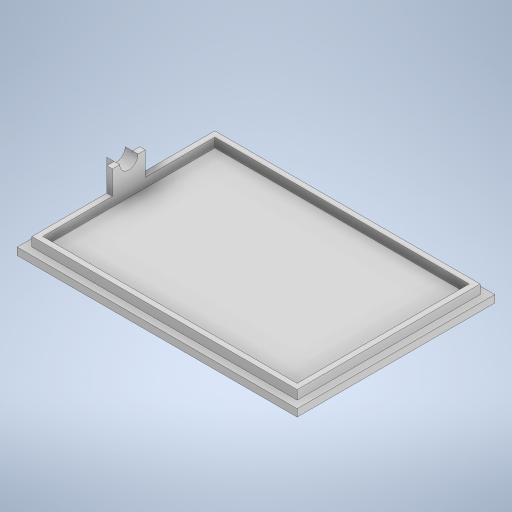
# Autodesk Inventor part: Golf Cart Mainboard Lid
Saved by Autodesk Inventor 2024 (Build 280153000, 153)
## iProperties
Created: 2023-08-08
Part Number: Golf Cart Mainboard Lid
Material: Generic
Document SubType Name: Modeling
Designer: techn
Density: 1 g/cm^3
Appearance: Default
Author: techn
## iProperties of the stored document Golf Cart Mainboard Lid_3DPrint.ipt
Created: 2023-08-08
Part Number: Golf Cart Mainboard Lid_3DPrint
Material: Generic
Document SubType Name: Modeling
Designer: techn
Density: 1 g/cm^3
Appearance: Default
Author: techn
Autodesk Inventor part; units mm, degrees
ref_plane "YZ Plane" through (0, 0, 0) normal (1, 0, 0) x (0, 1, 0)
ref_plane "XZ Plane" through (0, 0, 0) normal (0, 1, 0) x (-1, 0, 0)
ref_plane "XY Plane" through (0, 0, 0) normal (0, 0, 1) x (1, 0, 0)
sketch "Sketch1" plane through (0, 0, 0) normal (0, 1, 0) x (-1, 0, 0)
  line L0 (0, 0) -> (-153, 0)
  line L1 (-153, 0) -> (-153, 108)
  line L2 (-153, 108) -> (0, 108)
  line L3 (0, 108) -> (0, 0)
  dimension "d0" = 153
  dimension "d1" = 108
  constraints: 8 end point, 2 parallel, 1 horizontal, 1 perpendicular
  measures "d0" distance of L1.end L2.end
  measures "d1" distance of L0.end L1.end
extrude "Extrusion1" add sketch "Sketch1" along normal blind 4
sketch "Sketch2" plane through (0, 4, 0) normal (0, 1, 0) x (1, 0, 0)
  line L0 (0, -108) -> (153, -108) projected
  line L1 (0, -108) -> (4, -108)
  line L2 (4, -108) -> (4, -104)
  line L3 (4, -104) -> (0, -104)
  line L4 (0, -104) -> (0, -108)
  line L5 (4, -104) -> (149, -104)
  line L6 (149, -104) -> (149, -4)
  line L7 (149, -4) -> (4, -4)
  line L8 (4, -4) -> (4, -104)
  line L9 (153, -108) -> (153, 0) projected
  line L10 (0, -108) -> (153, -108)
  line L11 (153, -108) -> (153, 0)
  line L12 (153, 0) -> (0, 0)
  line L13 (0, 0) -> (0, -108)
  line L14 (4, -104) -> (7, -104)
  line L15 (7, -104) -> (7, -101)
  line L16 (7, -101) -> (4, -101)
  line L17 (4, -101) -> (4, -104)
  line L18 (7, -101) -> (146, -101)
  line L19 (146, -101) -> (146, -7)
  line L20 (146, -7) -> (7, -7)
  line L21 (7, -7) -> (7, -101)
  dimension "d4" = 4
  dimension "d5" = 4
  dimension "d6" = 145
  dimension "d7" = 100
  dimension "d8" = 3
  dimension "d9" = 3
  dimension "d10" = 139
  dimension "d11" = 94
  constraints: 40 end point, 10 parallel, 5 horizontal, 5 perpendicular
  measures "d4" distance of L3.end L2.end
  measures "d5" distance of L2.end L1.end
  measures "d6" distance of L7.end L6.end
  measures "d7" distance of L6.end L5.end
  measures "d8" distance of L16.end L15.end
  measures "d9" distance of L15.end L14.end
  measures "d10" distance of L20.end L19.end
  measures "d11" distance of L19.end L18.end
extrude "Extrusion2" add sketch "Sketch2" along normal blind 5 contours L8 L16 L15 L5 | L15 L16 L8 L7 L6 L5
sketch "Sketch3" plane through (0, 4, 0) normal (0, 1, 0) x (1, 0, 0)
  line L0 (0, 0) -> (0, -108) projected
  line L1 (0, -59) -> (4, -59)
  line L2 (4, -59) -> (4, -49)
  line L3 (4, -49) -> (0, -49)
  line L4 (0, -49) -> (0, -59)
  dimension "d14" = 4
  dimension "d15" = 10
  constraints: 8 end point, 2 parallel, 1 horizontal, 1 perpendicular, 1 point on line
  measures "d14" distance of L3.end L2.end
  measures "d15" distance of L2.end L1.end
extrude "Extrusion3" add sketch "Sketch3" along normal blind 18
sketch "Sketch4" plane through (4, 9, 49) normal (1, 0, 0) x (0, 0, -1)
  line L0 (0, 13) -> (-10, 13) projected
  circle A0 centre (-5, 13) radius 5
  point P0 (49, -9)
  constraints: 1 midpoint, 3 other
extrude "Extrusion4" cut sketch "Sketch4" against normal blind 18 contours A0 L0 picked at (-6.2475, 11.0971)
sketch "Sketch5" plane through (0, 9, 0) normal (0, 1, 0) x (1, 0, 0)
  line L0 (7, -101) -> (7, -7) projected
  line L1 (4, -45) -> (7, -45)
  line L2 (7, -45) -> (7, -63)
  line L3 (7, -63) -> (4, -63)
  line L4 (4, -63) -> (4, -45)
  point P0 (0, 0)
  dimension "d20" = 18
  constraints: 8 end point, 2 parallel, 1 horizontal, 1 perpendicular, 1 point on line
  measures "d20" distance of L1.end L2.end
extrude "Extrusion5" add sketch "Sketch5" along normal blind 13
sketch "Sketch6" plane through (4, 22, 54) normal (-1, 0, 0) x (0, 0, 1)
  line L0 (-5, 0) -> (5, 0) projected
  circle A0 centre (0, 0) radius 5
  point P0 (-54, -22)
  constraints: 1 midpoint, 3 other
extrude "Extrusion6" cut sketch "Sketch6" against normal blind 13 contours L0 A0 picked at (0.9468, -1.3716)
body "Solid1"
